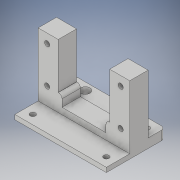
# Autodesk Inventor part: 30_CUBE_openSIM_DMD_Fixation_base
Saved by Autodesk Inventor 2019 (Build 230136000, 136)
## iProperties
Created: 2020-08-18
Part Number: 30_CUBE_openSIM_DMD_Fixation_base
Material: Generic
Document SubType Name: Modeling
Designer: wanghaoran
Density: 1 g/cm^3
Appearance: Default
Author: wanghaoran
Autodesk Inventor part; units mm, degrees
ref_plane "YZ Plane" through (0, 0, 0) normal (1, 0, 0) x (0, 1, 0)
ref_plane "XZ Plane" through (0, 0, 0) normal (0, 1, 0) x (-1, 0, 0)
ref_plane "XY Plane" through (0, 0, 0) normal (0, 0, 1) x (1, 0, 0)
sketch "Sketch1" plane through (0, 0, 0) normal (0, 0, 1) x (1, 0, 0)
  line L0 (0, 0) -> (49.8, 0)
  line L1 (49.8, 0) -> (49.8, 36.921)
  line L2 (49.8, 36.921) -> (0, 36.921)
  line L3 (0, 36.921) -> (0, 0)
  dimension "d0" = 49.8
  dimension "d1" = 36.921
  constraints: 8 end point, 2 parallel, 1 horizontal, 1 perpendicular
  measures "d0" distance of L2.end L1.end
  measures "d1" distance of L1.end L0.end
extrude "Extrusion1" add sketch "Sketch1" along normal blind 5
sketch "Sketch2" plane through (0, 0, 0) normal (0, 0, -1) x (-1, 0, 0)
  line L0 (0, 0) -> (-49.8, 0) projected
  line L1 (0, 0) -> (-49.8, 0)
  line L2 (-49.8, 0) -> (-49.8, 5)
  line L3 (-49.8, 5) -> (0, 5)
  line L4 (0, 5) -> (0, 0)
  dimension "d4" = 49.8
  dimension "d5" = 5
  constraints: 8 end point, 2 parallel, 1 horizontal, 1 perpendicular
  measures "d4" distance of L2.end L3.end
  measures "d5" distance of L1.end L2.end
extrude "Extrusion2" add sketch "Sketch2" along normal blind 30
sketch "Sketch4" plane through (0, 0, 0) normal (0, 0, -1) x (-1, 0, 0)
  line L0 (-38.9, 36.921) -> (-10.9, 36.921)
  line L1 (-10.9, 36.921) -> (-10.9, 12)
  line L2 (-10.9, 12) -> (-38.9, 12)
  line L3 (-38.9, 12) -> (-38.9, 36.921)
  line L4 (0, 36.921) -> (0, 5) projected
  line L5 (0, 5) -> (-49.8, 5) projected
  point P0 (0, 0)
  dimension "d24" = 28
  dimension "d25" = 24.921
  dimension "d26" = 10.9
  dimension "d27" = 7
  constraints: 8 end point, 2 parallel, 1 horizontal, 1 perpendicular
  measures "d24" distance of L1.end L2.end
  measures "d25" distance of L0.end L1.end
  measures "d26" distance between parallel lines of L4 L1
  measures "d27" distance between parallel lines of L5 L2
extrude "Extrusion3" cut sketch "Sketch4" against normal through all
sketch "Sketch6" plane through (0, 5, 0) normal (0, 1, 0) x (1, 0, 0)
  line L0 (0, -32.5) -> (49.8, -32.5)
  line L1 (49.8, -32.5) -> (49.8, 17.3)
  line L2 (49.8, 17.3) -> (0, 17.3)
  line L3 (0, 17.3) -> (0, -32.5)
  circle A0 centre (44.9, 9.4) radius 1.45
  circle A1 centre (4.9, 9.4) radius 1.45
  line L4 (24.9, 17.3) -> (24.9, 7.3)
  circle A2 centre (45.7, 3.9) radius 2.55
  circle A3 centre (39.4, 10.2) radius 2.55
  circle A4 centre (4.1, 3.9) radius 2.55
  circle A5 centre (10.4, 10.2) radius 2.55
  line L5 (49.8, 0) -> (49.8, 30) projected
  line L6 (0, 17.3) -> (49.8, 17.3)
  line L7 (49.8, 17.3) -> (49.8, 30)
  line L8 (49.8, 30) -> (0, 30)
  line L9 (0, 30) -> (0, 17.3)
  line L10 (49.8, 30) -> (49.8, -5) projected
  line L11 (0, 17.3) -> (49.8, 17.3)
  line L12 (49.8, 17.3) -> (49.8, 14.3)
  line L13 (49.8, 14.3) -> (0, 14.3)
  line L14 (0, 14.3) -> (0, 17.3)
  point P0 (0, 0)
  dimension "d36" = 49.8
  dimension "d37" = 49.8
  dimension "d38" = 2.9
  dimension "d39" = 4.9
  dimension "d40" = 7.9
  dimension "d41" = 2.9
  dimension "d42" = 4.9
  dimension "d43" = 7.9
  dimension "d44" = 10
  dimension "d45" = 5.1
  dimension "d46" = 5.1
  dimension "d47" = 4.1
  dimension "d48" = 13.4
  dimension "d49" = 10.4
  dimension "d50" = 7.1
  dimension "d64" = 3
  constraints: 26 end point, 6 centre point, 6 parallel, 3 horizontal, 3 perpendicular, 2 symmetric about line, 1 midpoint, 1 point on line, 1 vertical, 2 other
  measures "d36" distance of L2.end L1.end
  measures "d37" distance of L1.end L0.end
  measures "d38" diameter of A0
  measures "d39" distance from line of L1 A0.centre
  measures "d40" distance from line of L2 A0.centre
  measures "d41" diameter of A1
  measures "d42" distance from line of L3 A1.centre
  measures "d43" distance from line of L2 A1.centre
  measures "d44" distance of L4.start L4.end
  measures "d45" diameter of A2
  measures "d46" diameter of A3
  measures "d47" distance from line of L1 A2.centre
  measures "d48" distance from line of L2 A2.centre
  measures "d49" distance from line of L1 A3.centre
  measures "d50" distance from line of L2 A3.centre
  measures "d64" distance of L11.end L12.end
extrude "Extrusion5" cut sketch "Sketch6" against normal through all contours L3 L2 L4 L13 | L9 L8 L5 L2 | L4 L2 L1 L13 | A0 | A1 | A2 | A3 | A4 | A5
sketch "Sketch8" plane through (0, 0, 5) normal (0, 0, 1) x (1, 0, 0)
  line L0 (0, 0) -> (49.8, 0) projected
  line L1 (0, 0) -> (49.8, 0)
  line L2 (49.8, 0) -> (49.8, 2.5)
  line L3 (49.8, 2.5) -> (0, 2.5)
  line L4 (0, 2.5) -> (0, 0)
  dimension "d53" = 2.5
  constraints: 8 end point, 2 parallel, 1 horizontal, 1 perpendicular
  measures "d53" distance of L2.end L1.end
extrude "Extrusion6" add sketch "Sketch8" along normal blind 12.7
sketch "Sketch9" plane through (0, 2.5, 5) normal (0, 1, 0) x (1, 0, 0)
  circle A0 centre (44.9, -7.8) radius 1.45
  circle A1 centre (4.9, -7.8) radius 1.45
  line L0 (0, 0) -> (0, -12.7) projected
  line L1 (49.8, -12.7) -> (0, -12.7) projected
  line L2 (49.8, 0) -> (49.8, -12.7) projected
  point P0 (0, 5)
  dimension "d56" = 2.9
  dimension "d57" = 2.9
  dimension "d58" = 4.9
  dimension "d59" = 4.9
  dimension "d60" = 4.9
  dimension "d61" = 4.9
  constraints: 2 centre point
  measures "d56" diameter of A0
  measures "d57" diameter of A1
  measures "d58" distance from line of L0 A1.centre
  measures "d59" distance from line of L1 A1.centre
  measures "d60" distance from line of L1 A0.centre
  measures "d61" distance from line of L2 A0.centre
extrude "Extrusion7" cut sketch "Sketch9" against normal through all
fillet "Fillet1" radius 2 2 edges at (49.8, 2.5, -14.3) (0, 2.5, -14.3)
sketch "Sketch10" plane through (0, 0, 0) normal (0, 0, -1) x (-1, 0, 0)
  line L0 (-10.9, 36.921) -> (-10.9, 12) projected
  line L1 (-10.9, 12) -> (-38.9, 12) projected
  line L2 (-38.9, 12) -> (-38.9, 36.921) projected
  line L3 (-49.8, 36.921) -> (-38.9, 36.921) projected
  line L4 (-49.8, 5) -> (-49.8, 36.921) projected
  line L5 (-49.8, 5) -> (0, 5) projected
  line L6 (0, 36.921) -> (0, 5) projected
  line L7 (-10.9, 36.921) -> (0, 36.921) projected
  line L8 (-10.9, 18.4272) -> (-10.9, 27.6034)
  point P0 (0, 0)
  constraints: 2 end point, 1 vertical
extrude "Extrusion8" add sketch "Sketch10" along normal blind 5
sketch "Sketch3" plane through (0, 0, 0) normal (0, 0, -1) x (-1, 0, 0)
  circle A0 centre (-44.9, 31.921) radius 1.4
  circle A1 centre (-4.9, 31.921) radius 1.4
  circle A2 centre (-4.9, 12) radius 1.4
  line L0 (-49.8, 5) -> (-49.8, 36.921) projected
  line L1 (-49.8, 36.921) -> (0, 36.921) projected
  line L2 (0, 36.921) -> (0, 5) projected
  line L3 (0, 5) -> (-49.8, 5) projected
  circle A3 centre (-44.9, 12) radius 1.4
  point P0 (0, 0)
  dimension "d8" = 2.8
  dimension "d9" = 2.8
  dimension "d10" = 2.8
  dimension "d11" = 4.9
  dimension "d12" = 5
  dimension "d13" = 5
  dimension "d14" = 4.9
  dimension "d15" = 4.9
  dimension "d16" = 7
  dimension "d30" = 2.8
  dimension "d31" = 4.9
  dimension "d32" = 7
  constraints: 4 centre point
  measures "d8" diameter of A0
  measures "d9" diameter of A1
  measures "d10" diameter of A2
  measures "d11" distance from line of L0 A0.centre
  measures "d12" distance from line of L1 A0.centre
  measures "d13" distance from line of L1 A1.centre
  measures "d14" distance from line of L2 A1.centre
  measures "d15" distance from line of L2 A2.centre
  measures "d16" distance from line of L3 A2.centre
  measures "d30" diameter of A3
  measures "d31" distance from line of A3.centre L0
  measures "d32" distance from line of L3 A3.centre
extrude "Extrusion9" cut sketch "Sketch3" against normal blind 5 and the other way blind 5 contours A0 | A1 | A2 | A3
sketch "Sketch11" plane through (0, 0, -5) normal (0, 0, -1) x (-1, 0, 0)
  circle A0 centre (-44.9, 31.921) radius 1.4 projected
  circle A1 centre (-44.9, 31.921) radius 3
  circle A2 centre (-44.9, 12) radius 1.4 projected
  circle A3 centre (-44.9, 12) radius 3
  circle A4 centre (-4.9, 31.921) radius 1.4 projected
  circle A5 centre (-4.9, 31.921) radius 3
  circle A6 centre (-4.9, 12) radius 1.4 projected
  circle A7 centre (-4.9, 12) radius 3
  point P0 (0, 0)
  dimension "d72" = 6
  dimension "d73" = 6
  dimension "d74" = 6
  dimension "d75" = 6
  constraints: 4 centre point, 4 coincident
  measures "d72" diameter of A1
  measures "d73" diameter of A3
  measures "d74" diameter of A5
  measures "d75" diameter of A7
extrude "Extrusion10" cut sketch "Sketch11" against normal blind 2
sketch "Sketch12" plane through (0, 0, 5) normal (0, 0, 1) x (1, 0, 0)
  line L0 (38.9, 12) -> (10.9, 12) projected
  line L1 (13, 12) -> (36.9, 12)
  line L2 (36.9, 12) -> (36.9, 6)
  line L3 (36.9, 6) -> (13, 6)
  line L4 (13, 6) -> (13, 12)
  point P0 (0, 0)
  dimension "d78" = 23.9
  dimension "d79" = 6
  constraints: 8 end point, 2 parallel, 1 horizontal, 1 perpendicular, 1 point on line
  measures "d78" distance of L2.end L3.end
  measures "d79" distance of L1.end L2.end
extrude "Extrusion11" cut sketch "Sketch12" against normal blind 10
fillet "Fillet2" radius 2 2 edges at (13, 12, 0) (36.9, 12, 0)
body "Solid1"
